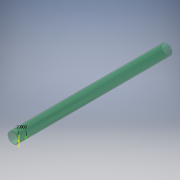
# Autodesk Inventor part: 2_5-inch schedule 40 forArm
Saved by Autodesk Inventor 2018.2 (Build 222227000, 227)
## iProperties
Created: 2018-01-07
Part Number: 2_5-inch schedule 40 forArm
Material: PVC-Piping
Document SubType Name: Modeling
Designer: steele
Density: 1.4 g/cm^3
Appearance: Clear - Green 1
Mass: 1559.84 g
Surface Area: 4359.5 cm^2
Volume: 1114.17 cm^3
Author: steele
Autodesk Inventor part; units mm, degrees
ref_plane "XZ Plane" through (0, 0, 0) normal (0, 1, 0) x (-1, 0, 0)
sketch "Sketch1" plane through (0, 0, 0) normal (0, 0, 1) x (1, 0, 0)
  circle A0 centre (0, 0) radius 31.3563
  circle A1 centre (0, 0) radius 36.5125
  dimension "d0" = 62.7126
  dimension "d1" = 73.025
  constraints: 2 centre point, 2 coincident
  measures "d0" diameter of A0
  measures "d1" diameter of A1
extrude "Extrusion1" add sketch "Sketch1" against normal blind 1016
ref_plane "Work Plane1" through (36.5125, 0, 0) normal (1, 0, 0) x (0, 1, 0)
sketch "Sketch2" plane through (36.5125, 0, 0) normal (1, 0, 0) x (0, 1, 0)
  circle A0 centre (0, -50.8) radius 23.8125 construction
  point P0 (0, 0)
  point P1 (0, -26.9875)
  point P2 (-20.6222, -38.8937)
  point P3 (-20.6222, -62.7062)
  point P4 (0, -74.6125)
  point P5 (20.6222, -62.7063)
  point P6 (20.6222, -38.8938)
  dimension "d4" = 47.625
  dimension "d5" = 50.8
  dimension "d8" = 360
  constraints: 2 coincident, 1 vertical alignment, 13 other
  measures "d5" distance of point (0, -50.8) point (0, 0)
hole "Hole1" at (36.5125, 0, -26.9875) at (36.5125, -20.6222, -38.8937) at (36.5125, -20.6222, -62.7062) at (36.5125, 0, -74.6125) at (36.5125, 20.6222, -62.7063) at (36.5125, 20.6222, -38.8938) direction (-1, 0, 0) diameter 5.1054 end through all clearance for "Flat Head Machine Screw (82)" size "#10" standard "Ansi Unified Screw Threads"
sketch "Sketch3" plane through (36.5125, 0, 0) normal (1, 0, 0) x (0, 1, 0)
  line L0 (-36.5125, 0) -> (36.5125, 0) projected
  point P0 (0, 0)
  point P1 (0, -50.8)
  dimension "d17" = 50.8
  measures "d17" distance from line of point (0, -50.8) L0
hole "Hole2" at (36.5125, 0, -50.8) direction (-1, 0, 0) diameter 12.7 end through all
ref_plane "Work Plane2" through (-36.5125, 0, 0) normal (1, 0, 0) x (0, 1, 0)
body "Solid1"
